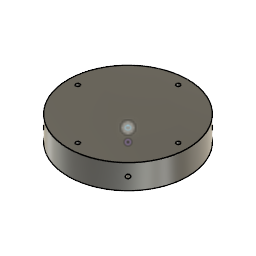
tank holder (Autodesk Fusion 360 design; units mm, degrees)
part number: 2026-03-31-20-17-39-117
Autodesk Fusion 360 part; units mm, degrees
sketch "Sketch1" plane through (0, 0, 0) normal (0, 0, 1) x (1, 0, 0)
  circle A0 centre (0, 0) radius 74.6125
  circle A1 centre (0, 62.7602) radius 2.4447
  line L0 (0, 74.6125) -> (0, -74.6125) construction
  line L1 (-74.6125, 0) -> (74.6125, 0) construction
  circle A2 centre (0, -62.7602) radius 2.4447
  circle A3 centre (-62.7602, 0) radius 2.4447
  circle A4 centre (62.7602, 0) radius 2.4447
  circle A5 centre (0, 0) radius 52.867
  dimension "d1" = 149.225
  dimension "d2" = 4.8895
  dimension "d3" = 4.8895
  dimension "d4" = 62.7602
  dimension "d5" = 62.7602
  constraint coincident A0.centre A5.centre
  constraint coincident A0 L0.start
  constraint coincident A0 L0.end
  constraint vertical L0
  constraint coincident A0 L1.start
  constraint coincident A0 L1.end
  constraint perpendicular L0 L1
  constraint coincident A1.centre L0
  constraint symmetric A1 L1 A2
  constraint coincident L1 A3.centre
  constraint symmetric L0 A3 A4
  measures "d1" diameter of A0
  measures "d2" diameter of A1
  measures "d3" diameter of A3
  measures "d4" distance of A0.centre A1.centre
  measures "d5" distance of A0.centre A3.centre
extrude "Extrude1" add sketch "Sketch1" along normal blind 30.48 contours A0 | A1 | A2 | A3 | A4 | A5
extrude "Extrude2" cut sketch "Sketch1" along normal blind 30.48 contours A1 | A2 | A3 | A4
ref_plane "WorkPlane1" through (0, 0, 12.125) normal (-0.707107, 0.707107, 0) x (0, 0, 1)
sketch "Sketch3" plane through (0, 0, 0) normal (-0.707107, 0.707107, 0) x (0, 0, 1)
  circle A0 centre (15.5211, 0) radius 2.4447
  dimension "d12" = 4.8895
  dimension "d29" = 15.5211
  measures "d12" diameter of A0
  measures "d29" distance of origin A0.centre
extrude "Extrude3" cut sketch "Sketch3" along normal blind 63.5 from surface at 44.1325
extrude "Extrude4" cut sketch "Sketch3" against normal blind 63.5 from surface at -44.1325
ref_plane "WorkPlane2" through (0, 0, 12.125) normal (-0.707107, -0.707107, 0) x (0, 0, 1)
sketch "Sketch4" plane through (0, 0, 0) normal (-0.707107, -0.707107, 0) x (0, 0, 1)
  circle A0 centre (15.551, 0.1414) radius 2.4447
  dimension "d20" = 4.8895
  measures "d20" diameter of A0
extrude "Extrude5" cut sketch "Sketch4" along normal blind 63.5 from surface at 44.1325
extrude "Extrude6" cut sketch "Sketch4" against normal blind 63.5 from surface at -44.1325
extrude "Extrude7" cut sketch "Sketch1" along normal blind 20.32 contours A5
